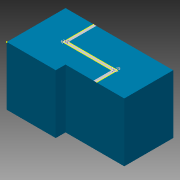
# Autodesk Inventor part: River 2_赤
Saved by Autodesk Inventor 2015 (Build 190159000, 159)
## iProperties
Created: 2015-08-24
Part Number: River 2_赤
Material: 一般
Document SubType Name: Modeling
Designer: nobuhiro
Density: 1 g/cm^3
Appearance: スカイ ブルー 標準
Author: nobuhiro
Autodesk Inventor part; units mm, degrees
ref_plane "YZ Plane" through (0, 0, 0) normal (1, 0, 0) x (0, 1, 0)
ref_plane "XZ Plane" through (0, 0, 0) normal (0, 1, 0) x (-1, 0, 0)
ref_plane "XY Plane" through (0, 0, 0) normal (0, 0, 1) x (1, 0, 0)
sketch "スケッチ1" plane through (0, 0, 0) normal (0, 0, 1) x (1, 0, 0)
  line L0 (0, 0) -> (0, 600)
  line L1 (0, 600) -> (1100, 600)
  line L2 (1100, 600) -> (1100, 100)
  line L3 (1100, 100) -> (500, 100)
  line L4 (500, 100) -> (500, 0)
  line L5 (500, 0) -> (0, 0)
  line L6 (285, 600) -> (315, 600)
  line L7 (315, 600) -> (315, 285)
  line L8 (315, 285) -> (285, 285)
  line L9 (285, 285) -> (285, 600)
  line L10 (285, 285) -> (815, 285)
  line L11 (815, 285) -> (815, 315)
  line L12 (815, 315) -> (285, 315)
  line L13 (285, 315) -> (285, 285)
  line L14 (785, 100) -> (815, 100)
  line L15 (815, 100) -> (815, 315)
  line L16 (815, 315) -> (785, 315)
  line L17 (785, 315) -> (785, 100)
  point P0 (285, 300)
  point P1 (0, 300)
  point P2 (800, 100)
  point P3 (800, 100)
  dimension "d0" = 600
  dimension "d1" = 1100
  dimension "d2" = 500
  dimension "d3" = 600
  dimension "d4" = 100
  dimension "d5" = 30
  dimension "d6" = 285
  constraints: 36 end point, 9 perpendicular, 6 parallel, 4 midpoint, 3 horizontal, 1 coincident, 1 horizontal alignment, 1 point on line, 1 vertical
  measures "d0" distance of L0.start L0.end
  measures "d1" distance of L0.end L1.end
  measures "d2" distance of L1.end L2.end
  measures "d3" distance of L2.end L3.end
  measures "d4" distance of L3.end L4.end
  measures "d5" distance between parallel lines of L9 L7
  measures "d6" distance between parallel lines of L9 L0
extrude "押し出し1" add sketch "スケッチ1" along normal blind 600 contours L0 L1 L9 L8 L10 L17 L3 L4 L5 | L1 L2 L3 L15 L11 L12 L7
sketch "スケッチ2" plane through (0, 0, 0) normal (0, 0, -1) x (-1, 0, 0)
  line L0 (-285, 285) -> (-785, 285) projected
  line L1 (-785, 285) -> (-785, 100) projected
  line L2 (-285, 600) -> (-285, 285) projected
  line L3 (-815, 315) -> (-315, 315) projected
  line L4 (-315, 315) -> (-315, 600) projected
  line L5 (-1100, 600) -> (-315, 600) projected
  line L6 (-1100, 100) -> (-1100, 600) projected
  line L7 (-815, 100) -> (-1100, 100) projected
  line L8 (-815, 100) -> (-815, 315) projected
  line L9 (-285, 600) -> (-315, 600)
  line L10 (-785, 100) -> (-815, 100)
  constraints: 4 end point, 1 horizontal, 1 parallel
extrude "押し出し2" add sketch "スケッチ2" against normal blind 600.1 contours L0 L1 L10 L8 L3 L4 L9 L2
sketch "スケッチ3" plane through (0, 0, 600.1) normal (0, 0, 1) x (1, 0, 0)
  line L0 (285, 600) -> (285, 285) projected
  line L1 (285, 285) -> (785, 285) projected
  line L2 (815, 100) -> (815, 315) projected
  line L3 (815, 315) -> (315, 315) projected
  point P0 (0, 0)
  point P1 (800, 300)
  point P2 (300, 300)
  dimension "d11" = 15
  dimension "d12" = 15
  dimension "d13" = 15
  dimension "d14" = 15
  measures "d11" distance from line of L0 point (300, 300)
  measures "d12" distance from line of point (300, 300) L1
  measures "d13" distance from line of point (800, 300) L2
  measures "d14" distance from line of point (800, 300) L3
equation "\"d12\" = d11"
equation "\"d14\" = d13"
